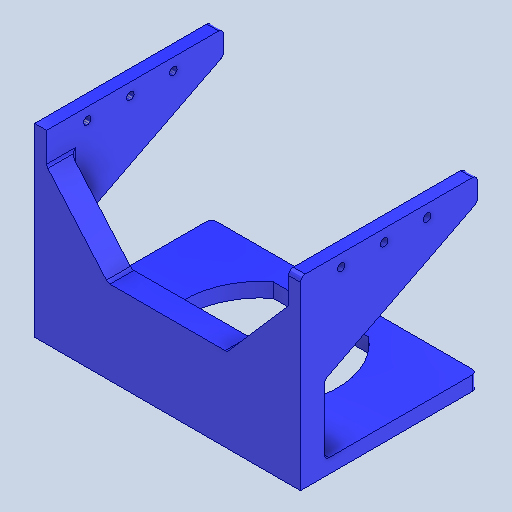
# Autodesk Inventor part: base_weel-v2-3DP-lidar-1
Saved by Autodesk Inventor 2025.2 (Build 292293000, 293)
## iProperties
Created: 2025-03-27
Part Number: base_weel-v2-3DP-lidar-1
Material: ABS プラスチック
Document SubType Name: Modeling
Designer: haruy
Density: 1.06 g/cm^3
Appearance: 青 - 壁塗料 - 光沢
Author: haruy
Autodesk Inventor part; units mm, degrees
ref_plane "YZ Plane" through (0, 0, 0) normal (1, 0, 0) x (0, 1, 0)
ref_plane "XZ Plane" through (0, 0, 0) normal (0, 1, 0) x (-1, 0, 0)
derived "base_weel-v2-Plate-7.ipt"
sketch "スケッチ1" plane through (0, 0, 0) normal (1, 0, 0) x (0, 1, 0)
  line L0 (0, 0) -> (20.1, 0)
  line L1 (20.1, 0) -> (20.1, -20)
  line L2 (20.1, -20) -> (0, -20)
  line L3 (0, -20) -> (0, 0)
  line L4 (0, -20) -> (5, -20)
  line L5 (5, -20) -> (5, -95)
  line L6 (5, -95) -> (0, -95)
  line L7 (0, -95) -> (0, -20)
  circle A0 centre (2.5, -38) radius 1.5 construction
  circle A1 centre (2.5, -56) radius 1.5 construction
  circle A2 centre (2.5, -74) radius 1.5 construction
  line L8 (20.1, 0) -> (25.1, 0)
  line L9 (25.1, 0) -> (25.1, -20)
  line L10 (25.1, -20) -> (20.1, -20)
  line L11 (20.1, -20) -> (20.1, 0)
  line L12 (0, 0) -> (-5, 0)
  line L13 (-5, 0) -> (-5, -20)
  line L14 (-5, -20) -> (0, -20)
  line L15 (0, -20) -> (0, 0)
  line L16 (25.1, -20) -> (5, -95)
  line L17 (-5, -20) -> (0, -95)
  line L18 (25.1, -25) -> (15.1, -25)
  line L19 (15.1, -25) -> (15.1, 0.1)
  line L20 (0, -25) -> (25.1, -25)
  line L21 (25.1, -25) -> (25.1, 0.1)
  line L22 (20.2704, -18.7057) -> (0.1704, -93.7057)
  line L23 (7, -95) -> (7, -18)
  line L24 (7, -18) -> (0, -18)
  line L25 (0, -35) -> (-35, -35)
  line L26 (-35, -35) -> (-35, -85)
  line L27 (-35, -85) -> (0, -85)
  line L28 (0, -85) -> (0, -35)
  line L29 (-35, -38) -> (-70, -38)
  line L30 (-70, -38) -> (-70, -82)
  line L31 (-70, -82) -> (-35, -82)
  line L32 (-35, -82) -> (-35, -38)
  line L33 (7.5, -95) -> (-2.5, -95)
  line L34 (-2.5, -95) -> (-2.5, -21)
  line L35 (-2.5, -21) -> (7.5, -21)
  line L36 (7.5, -21) -> (7.5, -95)
  line L37 (-2.5, -21) -> (-64, -21)
  line L38 (-64, -21) -> (-64, -31)
  line L39 (-64, -31) -> (-2.5, -31)
  line L40 (-2.5, -31) -> (-2.5, -21)
  circle A3 centre (2.5, -38) radius 1.6
  circle A4 centre (2.5, -56) radius 1.6
  circle A5 centre (2.5, -74) radius 1.6
  line L41 (-2.5, -95) -> (-35, -31)
  line L42 (-35, -31) -> (-35, -21)
  point P0 (0, -95)
  dimension "d1" = 3.2
  dimension "d2" = 3.2
  dimension "d3" = 3.2
  dimension "d4" = 0
  measures "d1" diameter of A3
  measures "d2" diameter of A4
  measures "d3" diameter of A5
  measures "d4" distance from line of L41.end L26
extrude "押し出し1" add sketch "スケッチ1" along normal blind 5 contours L35 L5 L20 L7 | L7 L25 L34 L35 | L37 L34 L39 L17 | L17 L39 L42 L37 | L35 L36 L20 L23 | L23 L20 L5 L35 | L36 L22 L23 L20 | L20 L5 L6 L7 | L39 L34 L25 L17 | L17 L25 L41 L39 | L42 L39 L38 L37 | L36 L16 L23 L22 | L23 L22 L5 L20 | L7 L27 L17 L34 L25 | L25 L34 L17 | L17 L34 L27 L41 L25 | L36 L33 L23 L16 | L23 L16 L5 L22 | L7 L17 L27 | L17 L27 L34 | L23 L33 L16 | L33 L34 L27 L17 | L34 L41 L27
extrude "押し出し2" add sketch "スケッチ1" against normal blind 101.2 contours L42 L39 L38 L37
ref_plane "作業平面1" through (-50.6, -64, -31) normal (-1, 0, 0) x (0, 0, 1)
mirror "ミラー1" about plane through (-50.6, -64, -31) normal (-1, 0, 0) of "押し出し1"
sketch "スケッチ2" plane through (5, -64, -31) normal (0, -1, 0) x (1, 0, 0)
  line L0 (-5, 10) -> (0, 10) projected
  line L1 (0, 10) -> (-111.2, 10)
  line L2 (-111.2, 10) -> (-111.2, -64)
  line L3 (-111.2, -64) -> (0, -64)
  line L4 (0, -64) -> (0, 10)
  line L5 (-5, -64) -> (0, -64) projected
  line L6 (-111.2, 0) -> (-111.2, -64) projected
  line L7 (0, -64) -> (-111.2, -64)
  line L8 (-111.2, -64) -> (-111.2, -54)
  line L9 (-111.2, -54) -> (0, -54)
  line L10 (0, -54) -> (0, -64)
  line L11 (-5, 0) -> (-106.2, 0) projected
  line L12 (-5, -54) -> (-106.2, -54)
  line L13 (-106.2, -54) -> (-106.2, 0)
  line L14 (-106.2, 0) -> (-5, 0)
  line L15 (-5, 0) -> (-5, -54)
  line L16 (-5, -54) -> (-5, -64)
  line L17 (-106.2, -54) -> (-106.2, -64)
  circle A0 centre (-55.5, -29) radius 22
  line L18 (-30.5, -4) -> (-80.5, -4)
  line L19 (-80.5, -4) -> (-80.5, -54)
  line L20 (-80.5, -54) -> (-30.5, -54)
  line L21 (-30.5, -54) -> (-30.5, -4)
  line L22 (-55.5, -29) -> (-55.5, -54)
  circle A1 centre (-55.5, -29) radius 32
  point P0 (-5, 31)
  point P1 (-41.9723, 0)
  point P2 (-35.525, -54)
  point P3 (-75.475, -54)
  point P4 (-69.0277, 0)
  dimension "d10" = 0
  dimension "d11" = 0
  dimension "d12" = 10
  dimension "d13" = 44
  dimension "d14" = 50
  dimension "d15" = 50
  dimension "d16" = 0
  dimension "d17" = 25
  dimension "d18" = 25
  dimension "d19" = 50.5
  dimension "d21" = 10
  constraints: 38 end point, 9 parallel, 4 horizontal, 4 perpendicular, 3 point on line, 2 centre point, 1 midpoint, 1 vertical
  measures "d10" distance between parallel lines of L5 L3
  measures "d11" distance between parallel lines of L6 L2
  measures "d12" distance of L7.end L8.end
  measures "d13" diameter of A0
  measures "d14" distance of L20.end L19.end
  measures "d15" distance of L19.end L18.end
  measures "d16" distance between parallel lines of L20 L12
  measures "d17" distance from line of L21 L22.start
  measures "d18" distance from line of L12 L22.start
  measures "d19" distance from line of L15 L22.start
  measures "d21" radial gap between concentric circles of A0 A1
extrude "押し出し3" add sketch "スケッチ2" along normal blind 6 contours L0 L4 L9 L15 L11 A1 L13 L2 L1 | L4 L3 L16 L9 | L16 L3 L17 L9 A1 | L9 L21 A1 L18 L11 L15 | L9 L17 L3 L2 | L9 A1 L21 | L13 L11 A1 L18 L19 L9 | A1 L9 | L11 A1 | L19 A1 L9 | A1 L18 L21 | A1 L19 L18
sketch "スケッチ3" plane through (-106.2, -70, -21) normal (0, 0, 1) x (1, 0, 0)
  line L0 (106.2, 35) -> (5, 35) projected
  line L1 (30.6, 35) -> (80.6, 35)
  line L2 (80.6, 35) -> (80.6, 70)
  line L3 (80.6, 70) -> (30.6, 70)
  line L4 (30.6, 70) -> (30.6, 35)
  line L5 (55.6, 70) -> (55.6, 35)
  line L6 (5, 77.5) -> (5, 35) projected
  line L7 (106.2, 77.5) -> (111.2, 77.5) projected
  line L8 (5, 77.5) -> (0, 77.5) projected
  line L9 (5, 64.5) -> (30.6, 35)
  line L10 (106.2, 64.5) -> (80.6, 35)
  line L11 (5, 64.5) -> (5, 35)
  line L12 (30.6, 35) -> (5, 35)
  line L13 (80.6, 35) -> (106.2, 35)
  line L14 (106.2, 35) -> (106.2, 64.5)
  point P0 (106.2, 70)
  point P1 (104, 35)
  point P2 (7, 35)
  point P3 (5, 75.5)
  point P4 (5, 37)
  point P5 (5.0615, 64.4288)
  dimension "d25" = 50
  dimension "d26" = 35
  dimension "d27" = 50.6
  dimension "d28" = 13
  constraints: 22 end point, 3 equal length, 2 midpoint, 2 perpendicular, 2 point on line, 1 horizontal, 1 symmetric about line, 1 vertical
  measures "d25" distance of L3.end L2.end
  measures "d26" distance of L2.end L1.end
  measures "d27" distance between parallel lines of L6 L5
  measures "d28" distance from line of L9.start L8
extrude "押し出し4" add sketch "スケッチ3" against normal blind 10 contours L0 L6 L9 | L0 L10 L14
fillet "フィレット2" radius 2 17 edges at (-101.2, -5.5, -26) (-75.6, -35, -26) (-25.6, -35, -26) (0, -5.5, -26) (2.5, 7.5, -21) (0, -20.25, -31) (2.5, -35, -31) (-101.2, -20.25, -31) (-103.7, -35, -31) (-85.1139, -64, -31) (-15.9861, -64, -31) (2.5, 7.5, -95) (2.5, -2.5, -95) (-103.7, 7.5, -95) (-103.7, -2.5, -95) (-106.2, -67, -95) (5, -67, -95)
equation "\"d18\" = d17"
